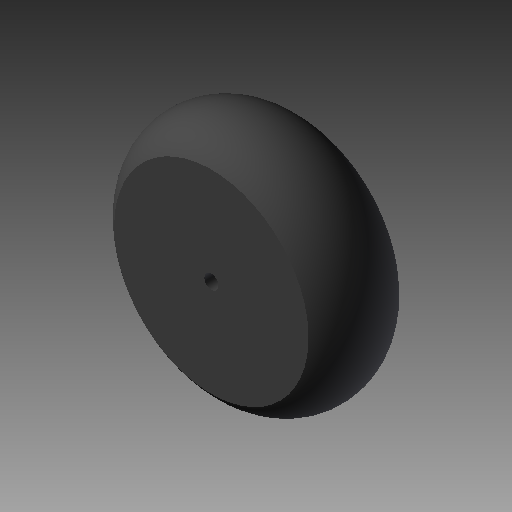
# Autodesk Inventor part: Llanta
Saved by Autodesk Inventor 2018 (Build 220112000, 112)
## iProperties
Created: 2020-01-19
Part Number: Llanta
Material: Generic
Document SubType Name: Modeling
Designer: peter
Density: 1 g/cm^3
Appearance: Default
Author: peter
Autodesk Inventor part; units mm, degrees
ref_plane "YZ Plane" through (0, 0, 0) normal (1, 0, 0) x (0, 1, 0)
ref_plane "XZ Plane" through (0, 0, 0) normal (0, 1, 0) x (-1, 0, 0)
ref_plane "XY Plane" through (0, 0, 0) normal (0, 0, 1) x (1, 0, 0)
sketch "Sketch1" plane through (0, 0, 0) normal (0, 1, 0) x (-1, 0, 0)
  line L0 (-58.5915, 19.6718) -> (-85.8369, 19.6718)
  line L1 (-58.5915, 44.6718) -> (-85.8369, 44.6718)
  line L2 (-85.8369, 19.6718) -> (-85.8369, 44.6718)
  line L3 (-83.8369, 19.6718) -> (-83.8369, 44.6718)
  arc A0 (-58.5915, 19.6718) -> (-58.5915, 44.6718) centre (-66.8831, 32.1718) ccw
  point P0 (0, 0)
  dimension "d2" = 27.2454
  dimension "d5" = 2
  dimension "d8" = 27.2454
  dimension "d12" = 25
  constraints: 8 end point, 2 point on circle, 2 point on line, 1 centre point, 1 horizontal, 1 parallel, 1 perpendicular, 1 vertical
  measures "d2" distance of L0.start L0.end
  measures "d5" distance of L1.end L3.end
  measures "d8" distance of L1.start L1.end
  measures "d12" distance of L0.end L1.end
revolve "Revolution1" add sketch "Sketch1" angle 360 about axis through (85.8369, 0, 19.6718) along (0, 0, 1) contours L0 L3 L1 A0
body "Solid1"
